Limit_switch support_v2 (Autodesk Fusion 360 design; units mm, degrees)
Autodesk Fusion 360 part; units mm, degrees
sketch "Esquisse5" plane through (0, 0, 0) normal (0, 0, 1) x (1, 0, 0)
  line L0 (16.9, -17.9) -> (-16.9, -17.9)
  line L1 (-16.9, -17.9) -> (-16.9, 17.9)
  line L2 (-16.9, 17.9) -> (16.9, 17.9)
  line L3 (16.9, 17.9) -> (16.9, -17.9)
  line L4 (16.9, -17.9) -> (-16.9, 17.9) construction
  line L5 (-16.9, -17.9) -> (16.9, 17.9) construction
  circle A0 centre (-13.9, -14.9) radius 1.7
  line L6 (0, 0) -> (0, -17.9) construction
  line L7 (0, 0) -> (16.9, 0) construction
  circle A1 centre (13.9, -14.9) radius 1.7
  circle A2 centre (-13.9, 14.9) radius 1.7
  circle A3 centre (13.9, 14.9) radius 1.7
  line L8 (10.8, 9.17) -> (-10.8, 9.17)
  line L9 (-10.8, 9.17) -> (-10.8, -9.17)
  line L10 (-10.8, -9.17) -> (10.8, -9.17)
  line L11 (10.8, -9.17) -> (10.8, 9.17)
  line L12 (10.8, 9.17) -> (-10.8, -9.17) construction
  line L13 (-10.8, 9.17) -> (10.8, -9.17) construction
  line L14 (-10.05, -3.25) -> (10.05, -3.25)
  line L15 (10.05, -3.25) -> (10.05, 3.25)
  line L16 (10.05, 3.25) -> (-10.05, 3.25)
  line L17 (-10.05, 3.25) -> (-10.05, -3.25)
  line L18 (-10.05, -3.25) -> (10.05, 3.25) construction
  line L19 (10.05, -3.25) -> (-10.05, 3.25) construction
  dimension "d54" = 33.8
  dimension "d55" = 35.8
  dimension "d56" = 3.4
  dimension "d57" = 3
  dimension "d58" = 3
  dimension "d59" = 21.6
  dimension "d60" = 18.34
  dimension "d61" = 20.1
  dimension "d62" = 6.5
  constraint horizontal L0
  constraint perpendicular L0 L1
  constraint parallel L0 L2
  constraint parallel L1 L3
  constraint coincident L4 L6.start
  constraint coincident L5 L6.start
  constraint coincident L6.start L7.start
  constraint midpoint L0 L6.end
  constraint midpoint L3 L7.end
  constraint symmetric A0 L6 A1
  constraint symmetric A0 L7 A2
  constraint symmetric L7 A1 A3
  constraint horizontal L8
  constraint perpendicular L8 L9
  constraint parallel L8 L10
  constraint parallel L9 L11
  constraint coincident L12 L6.start
  constraint coincident L13 L6.start
  constraint horizontal L14
  constraint perpendicular L14 L15
  constraint parallel L14 L16
  constraint parallel L15 L17
  constraint coincident L18 L6.start
  constraint coincident L19 L6.start
  measures "d54" distance of L1.end L2.end
  measures "d55" distance of L0.end L1.end
  measures "d56" diameter of A0
  measures "d57" distance of L0 A0.centre
  measures "d58" distance of L1 A0.centre
  measures "d59" distance of L9.end L10.end
  measures "d60" distance of L8.end L9.end
  measures "d61" distance of L15.end L16.end
  measures "d62" distance of L14.end L15.end
extrude "Extrusion3" add sketch "Esquisse5" against normal blind 3 contours L8 L9 L10 L11
extrude "Extrusion4" add sketch "Esquisse5" along normal blind 2 contours L0 L1 L2 L3
extrude "Extrusion5" add sketch "Esquisse5" along normal blind 7 contours L8 L9 L10 L11
sketch "Esquisse6" plane through (0, 9.17, 0) normal (0, 1, 0) x (-1, 0, 0)
  line L0 (-10.8, 2) -> (10.8, 2)
  line L1 (10.8, 2) -> (10.8, 7)
  line L2 (10.8, 7) -> (-10.8, 7)
  line L3 (-10.8, 7) -> (-10.8, 2)
  circle A0 centre (4.75, 3.75) radius 1.25
  circle A1 centre (-4.75, 3.75) radius 1.25
  line L4 (0, 2) -> (0, 7) construction
  dimension "d69" = 2.5
  dimension "d70" = 2.5
  dimension "d71" = 3.25
  dimension "d72" = 3.25
  dimension "d73" = 9.5
  constraint midpoint L0 L4.start
  constraint midpoint L2 L4.end
  constraint symmetric A0 A1 L4
  measures "d69" diameter of A0
  measures "d70" diameter of A1
  measures "d71" distance of L2 A0.centre
  measures "d72" distance of L2 A1.centre
  measures "d73" distance of A0.centre A1.centre
extrude "Extrusion6" cut sketch "Esquisse6" against normal through all contours A0 | A1
sketch "Esquisse7" plane through (0, 0, 7) normal (0, 0, 1) x (-1, 0, 0)
  line L0 (10.05, 3.25) -> (10.05, -3.25)
  line L1 (10.05, -3.25) -> (-10.05, -3.25)
  line L2 (-10.05, -3.25) -> (-10.05, 3.25)
  line L3 (-10.05, 3.25) -> (10.05, 3.25)
  line L4 (-10.8, 9.17) -> (-10.8, -9.17)
  line L5 (-10.8, -9.17) -> (10.8, -9.17)
  line L6 (10.8, -9.17) -> (10.8, 9.17)
  line L7 (10.8, 9.17) -> (-10.8, 9.17)
  line L8 (10.8, -6.25) -> (-10.8, -6.25)
  line L9 (-10.05, -3.25) -> (10.05, -3.25)
  line L10 (10.8, 6.25) -> (-10.8, 6.25)
  dimension "d76" = 3
  dimension "d77" = 3
  constraint coincident L6 L8.start
  constraint coincident L4 L8.end
  constraint perpendicular L4 L8
  constraint coincident L6 L10.start
  constraint coincident L4 L10.end
  constraint perpendicular L4 L10
  measures "d76" distance of L8 L9
  measures "d77" distance of L3 L10
extrude "Extrusion7" cut sketch "Esquisse7" against normal blind 5 contours L4 L6 L7 L10 | L4 L5 L6 L8
move_face "DécalerLesFaces1" offset 1 1 faces at (10.8, -2.0833, 3.6667)
move_face "DécalerLesFaces2" offset 1 1 faces at (-10.8, 2.0833, 3.6667)
equation "d70 = d69"
equation "d71 = 2 mm + ( 2.5 / 2 ) * 1 mm"
equation "d72 = d71"
equation "d73 = 7 mm + d69"
